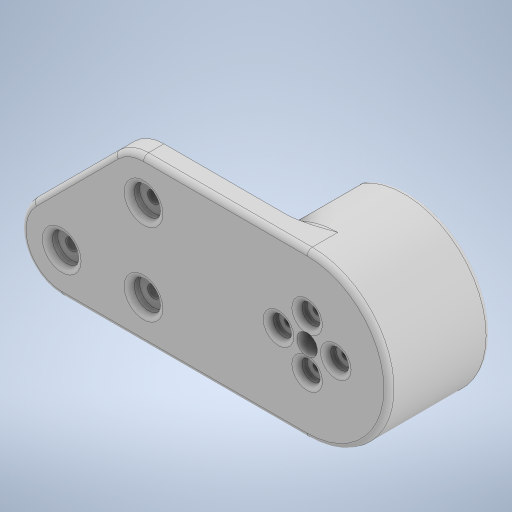
# Autodesk Inventor part: BLDC Bracket
Saved by Autodesk Inventor 2024 (Build 280153000, 153)
## iProperties
Created: 2024-01-19
Part Number: BLDC Bracket
Material: Generic
Document SubType Name: Modeling
Designer: CJ110
Density: 1 g/cm^3
Appearance: Default
Author: CJ110
Autodesk Inventor part; units mm, degrees
ref_plane "YZ Plane" through (0, 0, 0) normal (1, 0, 0) x (0, 1, 0)
ref_plane "XZ Plane" through (0, 0, 0) normal (0, 1, 0) x (-1, 0, 0)
ref_plane "XY Plane" through (0, 0, 0) normal (0, 0, 1) x (1, 0, 0)
sketch "Sketch1" plane through (0, 0, 0) normal (0, 0, 1) x (1, 0, 0)
  line L0 (0, 0) -> (114.3, 0)
  line L1 (114.3, 0) -> (114.3, 50.8)
  line L2 (114.3, 50.8) -> (0, 50.8)
  line L3 (0, 50.8) -> (0, 0)
  dimension "d0" = 114.3
  dimension "d1" = 50.8
  constraints: 8 end point, 2 parallel, 1 horizontal, 1 perpendicular
  measures "d0" distance between parallel lines of L3 L1
  measures "d1" distance between parallel lines of L0 L2
extrude "Extrusion1" add sketch "Sketch1" against normal blind 6.35
sketch "Sketch2" plane through (0, 0, 0) normal (0, 0, 1) x (1, 0, 0)
  line L0 (114.3, 0) -> (114.3, 50.8) projected
  line L1 (114.3, 50.8) -> (0, 50.8) projected
  line L2 (0, 50.8) -> (0, 0) projected
  line L3 (0, 0) -> (114.3, 0) projected
  line L4 (0, 25.4) -> (114.3, 25.4) construction
  circle A0 centre (12.7, 12.7) radius 1.905
  circle A1 centre (12.7, 12.7) radius 4.445
  circle A2 centre (38.1, 12.7) radius 1.905
  circle A3 centre (38.1, 12.7) radius 4.445
  circle A4 centre (38.1, 38.1) radius 1.905
  circle A5 centre (38.1, 38.1) radius 4.445
  line L5 (0, 17.9605) -> (32.8395, 50.8)
  line L6 (0, 0) -> (50.8, 50.8) construction
  circle A6 centre (38.1, 38.1) radius 12.7 construction
  dimension "d4" = 3.81
  dimension "d5" = 8.89
  dimension "d6" = 25.4
  dimension "d7" = 25.4
  dimension "d8" = 12.7
  dimension "d10" = 12.7
  constraints: 7 centre point, 6 end point, 4 coincident, 4 equal radius, 4 point on line, 2 midpoint, 2 tangent, 1 horizontal, 1 horizontal alignment, 1 parallel, 1 vertical alignment
  measures "d4" diameter of A4
  measures "d5" diameter of A5
  measures "d6" distance of A0.centre A2.centre
  measures "d7" distance of A2.centre A4.centre
  measures "d8" distance from line of L4 A0.centre
  measures "d10" distance from line of L2 A0.centre
extrude "Extrusion2" cut sketch "Sketch2" against normal through all contours L5 L2 L1 | A0 | A2 | A4
extrude "Extrusion3" cut sketch "Sketch2" against normal blind 3.175 contours A1 | A3 | A5
sketch "Sketch3" plane through (0, 0, 0) normal (0, 0, 1) x (1, 0, 0)
  circle A0 centre (88.9, 25.4) radius 3.175
  circle A1 centre (88.9, 33.02) radius 1.27
  circle A2 centre (88.9, 33.02) radius 3.175
  circle A3 centre (88.9, 17.78) radius 1.27
  circle A4 centre (88.9, 17.78) radius 3.175
  circle A5 centre (80.01, 25.4) radius 1.27
  circle A6 centre (80.01, 25.4) radius 3.175
  circle A7 centre (97.79, 25.4) radius 1.27
  circle A8 centre (97.79, 25.4) radius 3.175
  circle A9 centre (38.1, 12.7) radius 4.445 projected
  circle A10 centre (12.7, 12.7) radius 4.445 projected
  circle A11 centre (38.1, 38.1) radius 4.445 projected
  line L0 (32.8395, 50.8) -> (0, 17.9605) projected
  line L1 (0, 17.9605) -> (0, 0) projected
  line L2 (0, 0) -> (114.3, 0) projected
  line L3 (114.3, 0) -> (114.3, 50.8) projected
  line L4 (114.3, 50.8) -> (32.8395, 50.8) projected
  line L5 (114.3, 25.4) -> (7.4395, 25.4) construction
  dimension "d16" = 8.89
  dimension "d17" = 8.89
  dimension "d18" = 7.62
  dimension "d19" = 7.62
  dimension "d20" = 2.54
  dimension "d21" = 6.35
  dimension "d22" = 25.4
  constraints: 9 centre point, 7 equal radius, 4 coincident, 4 point on line, 2 end point, 2 vertical alignment, 1 horizontal, 1 midpoint
  measures "d16" distance of A7.centre A0.centre
  measures "d17" distance of A6.centre A0.centre
  measures "d18" distance of A3.centre A0.centre
  measures "d19" distance of A0.centre A1.centre
  measures "d20" diameter of A7
  measures "d21" diameter of A8
  measures "d22" distance from line of L3 A0.centre
extrude "Extrusion4" cut sketch "Sketch3" against normal through all contours A0 | A1 | A3 | A5 | A7
extrude "Extrusion5" cut sketch "Sketch3" against normal blind 3.175 contours A2 | A4 | A6 | A8
sketch "Sketch4" plane through (0, 0, -6.35) normal (0, 0, -1) x (-1, 0, 0)
  circle A0 centre (-88.9, 17.78) radius 1.27 projected
  circle A1 centre (-97.79, 25.4) radius 1.27 projected
  circle A2 centre (-80.01, 25.4) radius 1.27 projected
  circle A3 centre (-88.9, 25.4) radius 3.175 projected
  circle A4 centre (-88.9, 33.02) radius 1.27 projected
  line L0 (0, 17.9605) -> (-32.8395, 50.8) projected
  line L1 (-32.8395, 50.8) -> (-114.3, 50.8) projected
  line L2 (-114.3, 50.8) -> (-114.3, 0) projected
  line L3 (-114.3, 0) -> (0, 0) projected
  line L4 (0, 0) -> (0, 17.9605) projected
  circle A5 centre (-12.7, 12.7) radius 1.905 projected
  circle A6 centre (-38.1, 38.1) radius 1.905 projected
  circle A7 centre (-38.1, 12.7) radius 1.905 projected
  circle A8 centre (-88.9, 25.4) radius 25.4
  circle A9 centre (-88.9, 25.4) radius 19.05
  line L5 (-88.9, 25.4) -> (-76.2, 47.397)
  line L6 (-88.9, 25.4) -> (-76.2, 3.403)
  line L7 (-114.3, 25.4) -> (-63.5, 25.4) construction
  circle A10 centre (-77.7875, 44.6474) radius 3.175
  circle A11 centre (-77.7875, 6.1526) radius 3.175
  point P0 (-79.375, 8.9022)
  point P1 (-79.375, 41.8978)
  point P2 (-76.2, 3.403)
  point P3 (-79.375, 8.9022)
  point P4 (-79.375, 41.8978)
  point P5 (-76.2, 47.397)
  dimension "d27" = 38.1
  dimension "d28" = 60
  dimension "d29" = 60
  constraints: 6 end point, 5 tangent, 4 centre point, 4 point on circle, 2 coincident, 2 point on line, 1 midpoint, 1 perpendicular
  measures "d27" diameter of A9
  measures "d28" angle of L7 L5
  measures "d29" angle of L7 L6
extrude "Extrusion6" add sketch "Sketch4" along normal blind 25.4 contours A10 L5 | A9 A11 A8 A10 | L5 A10 | A11 L6 | L6 A11 picked at (-95.816, 47.4856)
sketch "Sketch5" plane through (0, 0, 0) normal (0, 0, 1) x (1, 0, 0)
  circle A0 centre (88.9, 17.78) radius 3.175 projected
  circle A1 centre (80.01, 25.4) radius 3.175 projected
  circle A2 centre (97.79, 25.4) radius 3.175 projected
  circle A3 centre (88.9, 33.02) radius 3.175 projected
  circle A4 centre (88.9, 25.4) radius 3.175 projected
  circle A5 centre (38.1, 12.7) radius 4.445 projected
  circle A6 centre (12.7, 12.7) radius 4.445 projected
  circle A7 centre (38.1, 38.1) radius 4.445 projected
  line L0 (32.8395, 50.8) -> (0, 17.9605) projected
  line L1 (0, 17.9605) -> (0, 0) projected
  line L2 (0, 0) -> (114.3, 0) projected
  line L3 (114.3, 0) -> (114.3, 50.8) projected
  line L4 (114.3, 50.8) -> (32.8395, 50.8) projected
  arc A8 (79.375, 8.9022) -> (79.375, 41.8978) centre (88.9, 25.4) ccw projected
  arc A9 (76.2, 3.403) -> (76.2, 47.397) centre (88.9, 25.4) ccw projected
  arc A10 (76.2, 47.397) -> (79.375, 41.8978) centre (77.7875, 44.6474) ccw projected
  arc A11 (79.375, 8.9022) -> (76.2, 3.403) centre (77.7875, 6.1526) ccw projected
  point P0 (114.3, 25.4)
  point P1 (88.9, 0)
  point P2 (88.9, 50.8)
extrude "Extrusion7" cut sketch "Sketch5" against normal through all contours L4 L3 A9 | L3 L2 A9
fillet "Fillet1" radius 1.5875 7 edges at (33.655, 38.1, 0) (8.255, 12.7, 0) (33.655, 12.7, 0) (85.725, 33.02, 0) (76.835, 25.4, 0) (85.725, 17.78, 0) (94.615, 25.4, 0)
sketch "Sketch6" plane through (0, 0, 0) normal (0, 0, 1) x (1, 0, 0)
  circle A0 centre (80.01, 25.4) radius 4.7625 projected
  circle A1 centre (12.7, 12.7) radius 6.0325 projected
  arc A2 (88.9, 0) -> (88.9, 50.8) centre (88.9, 25.4) ccw projected
  line L0 (88.9, 50.8) -> (32.8395, 50.8) projected
  line L1 (32.8395, 50.8) -> (0, 17.9605) projected
  line L2 (0, 17.9605) -> (0, 0) projected
  line L3 (0, 0) -> (88.9, 0) projected
  circle A3 centre (38.1, 38.1) radius 6.0325 projected
  circle A4 centre (38.1, 12.7) radius 6.0325 projected
  arc A5 (87.8131, 22.4168) -> (89.9869, 22.4168) centre (88.9, 17.78) ccw projected
  arc A6 (87.8131, 28.3832) -> (87.8131, 22.4168) centre (88.9, 25.4) ccw projected
  arc A7 (89.9869, 28.3832) -> (87.8131, 28.3832) centre (88.9, 33.02) ccw projected
  arc A8 (89.9869, 22.4168) -> (89.9869, 28.3832) centre (88.9, 25.4) ccw projected
  circle A9 centre (97.79, 25.4) radius 4.7625 projected
  circle A10 centre (12.7, 12.7) radius 12.7
  circle A11 centre (38.1, 38.1) radius 12.7
  line L4 (88.9, 50.8) -> (32.8395, 50.8) projected
  point P0 (0, 12.7)
  point P1 (3.7197, 21.6803)
  point P2 (12.7, 0)
  point P3 (29.1197, 47.0803)
  point P4 (38.1, 50.8)
  constraints: 2 centre point, 2 coincident, 2 tangent
extrude "Extrusion8" cut sketch "Sketch6" against normal through all contours L3 L2 A10 | A11 L1 L0 | L2 L1 A10
fillet "Fillet2" radius 1.5875 6 edges at (33.2399, 49.8333, 0) (16.4197, 34.3803, 0) (0.9667, 7.8399, 0) (50.8, 0, 0) (114.3, 25.4, 0) (63.5, 50.8, 0)
fillet "Fillet3" radius 3.175 5 edges at (75.0379, 7.7401, -6.35) (82.326, 49.9345, -6.35) (82.326, 0.8655, -6.35) (75.0379, 43.0599, -6.35) (107.95, 25.4, -6.35)
fillet "Fillet4" radius 1.5875 4 edges at (75.0379, 43.0599, -31.75) (114.3, 25.4, -31.75) (75.0379, 7.7401, -31.75) (107.95, 25.4, -31.75)
equation "\"d17\" = d16"
equation "\"d19\" = d18"
equation "\"d29\" = d28"
body "Solid1"
